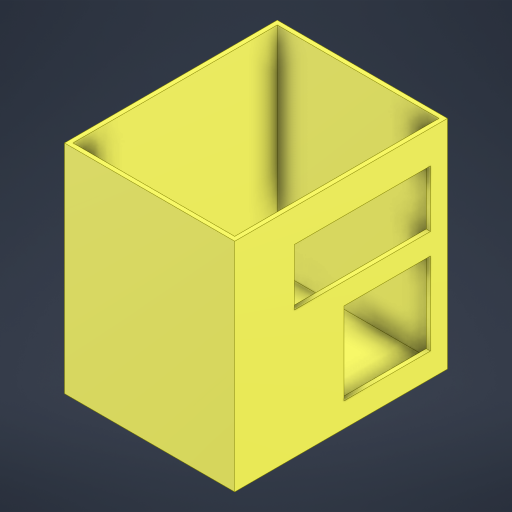
# Autodesk Inventor part: perspex_shell
Saved by Autodesk Inventor 2023 (Build 270158000, 158)
## iProperties
Created: 2022-11-19
Part Number: perspex_shell
Material: Generic
Document SubType Name: Modeling
Designer: washington
Density: 1 g/cm^3
Appearance: Smooth - Yellow
Author: washington
Autodesk Inventor part; units mm, degrees
ref_plane "YZ Plane" through (0, 0, 0) normal (1, 0, 0) x (0, 1, 0)
ref_plane "XZ Plane" through (0, 0, 0) normal (0, 1, 0) x (-1, 0, 0)
ref_plane "XY Plane" through (0, 0, 0) normal (0, 0, 1) x (1, 0, 0)
sketch "Sketch1" plane through (0, 0, 0) normal (0, 1, 0) x (-1, 0, 0)
  line L0 (60, 75) -> (-60, 75)
  line L1 (-60, 75) -> (-60, -75)
  line L2 (-60, -75) -> (60, -75)
  line L3 (60, -75) -> (60, 75)
  line L4 (60, 75) -> (-60, -75) construction
  line L5 (-60, 75) -> (60, -75) construction
  point P0 (0, 0)
  dimension "d0" = 150
  dimension "d1" = 120
  constraints: 12 end point, 2 midpoint, 2 parallel, 1 horizontal, 1 perpendicular
  measures "d0" distance of L0.end L1.end
  measures "d1" distance of L1.end L2.end
extrude "Extrusion1" add sketch "Sketch1" along normal blind 3
sketch "Sketch2" plane through (0, 3, 0) normal (0, 1, 0) x (1, 0, 0)
  line L0 (60, -75) -> (60, 75) projected
  line L1 (-60, -75) -> (60, -75)
  line L2 (60, -75) -> (60, 75)
  line L3 (60, 75) -> (-60, 75)
  line L4 (-60, 75) -> (-60, -75)
  line L5 (-60, -75) -> (60, 75) construction
  line L6 (60, -75) -> (-60, 75) construction
  line L7 (-57, -72) -> (57, -72)
  line L8 (57, -72) -> (57, 72)
  line L9 (57, 72) -> (-57, 72)
  line L10 (-57, 72) -> (-57, -72)
  line L11 (-57, -72) -> (57, 72) construction
  line L12 (57, -72) -> (-57, 72) construction
  point P0 (0, 0)
  point P1 (60, -75)
  dimension "d4" = 144
  dimension "d5" = 114
  constraints: 24 end point, 4 midpoint, 4 parallel, 2 horizontal, 2 perpendicular
  measures "d4" distance of L7.end L8.end
  measures "d5" distance of L8.end L9.end
extrude "Extrusion2" add sketch "Sketch2" along normal blind 150
sketch "Sketch3" plane through (60, 0, 75) normal (1, 0, 0) x (0, 0, -1)
  line L0 (42, 130) -> (138, 130)
  line L1 (138, 130) -> (138, 90)
  line L2 (138, 90) -> (42, 90)
  line L3 (42, 90) -> (42, 130)
  line L4 (42, 130) -> (138, 90) construction
  line L5 (138, 130) -> (42, 90) construction
  line L6 (0, 0) -> (0, 153) projected
  line L7 (77, 75) -> (138, 75)
  line L8 (138, 75) -> (138, 17)
  line L9 (138, 17) -> (77, 17)
  line L10 (77, 17) -> (77, 75)
  line L11 (77, 75) -> (138, 17) construction
  line L12 (138, 75) -> (77, 17) construction
  point P0 (75, 0)
  point P1 (90, 110)
  point P2 (107.5, 46)
  dimension "d8" = 96
  dimension "d9" = 40
  dimension "d10" = 90
  dimension "d11" = 110
  dimension "d14" = 61
  dimension "d15" = 58
  dimension "d16" = 0
  dimension "d17" = 46
  constraints: 24 end point, 4 midpoint, 4 parallel, 2 horizontal, 2 perpendicular
  measures "d8" distance of L1.end L2.end
  measures "d9" distance of L0.end L1.end
  measures "d10" distance from line of point (90, 110) L6
  measures "d11" vertical distance of point (90, 110) L6.start
  measures "d14" distance of L8.end L9.end
  measures "d15" distance of L7.end L8.end
  measures "d16" distance between parallel lines of L1 L8
  measures "d17" vertical distance of L6.start point (107.5, 46)
extrude "Extrusion3" cut sketch "Sketch3" against normal blind 3
body "Solid1"
